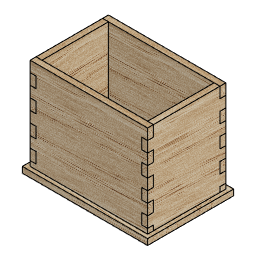
laser cut box_ (Autodesk Fusion 360 design; units mm, degrees)
Autodesk Fusion 360 part; units mm, degrees
sketch "base" plane through (0, 0, 0) normal (0, 0, 1) x (1, 0, 0) in component "base"
  line L0 (0, 0) -> (60, 0)
  line L1 (60, 0) -> (60, 40)
  line L2 (60, 40) -> (0, 40)
  line L3 (0, 40) -> (0, 0)
  line L4 (60, 20) -> (0, 20) construction
  line L5 (30, 40) -> (30, 0) construction
  line L6 (-2, 42) -> (62, 42)
  line L7 (62, 42) -> (62, -2)
  line L8 (62, -2) -> (-2, -2)
  line L9 (-2, -2) -> (-2, 42)
  line L10 (-2, 42) -> (62, -2) construction
  line L11 (62, 42) -> (-2, -2) construction
  point P0 (30, 20)
  dimension "d14" = 60
  dimension "d15" = 40
  dimension "d16" = 2
  dimension "d17" = 2
  constraint horizontal L0
  constraint vertical L1
  constraint horizontal L2
  constraint vertical L3
  constraint coincident L0.start L3.end
  constraint midpoint L1 L4.start
  constraint midpoint L3 L4.end
  constraint midpoint L2 L5.start
  constraint midpoint L0 L5.end
  constraint horizontal L6
  constraint perpendicular L6 L7
  constraint parallel L6 L8
  constraint parallel L7 L9
  constraint coincident L10 P0
  constraint coincident L11 P0
  constraint midpoint L4 P0
  measures "d14" distance of L1.end L2.end
  measures "d15" distance of L0.end L1.end
  measures "d16" distance of L2 L6
  measures "d17" distance of L1 L7
extrude "Extrude1" add sketch "base" along normal blind 3 contours L0 L1 L2 L3 | L6 L7 L8 L9 makes body 1 in component "base"
sketch "lenghttabcut" plane through (0, 0, 3) normal (0, 0, 1) x (-1, 0, 0) in component "base"
  line L0 (2, 2) -> (-62, 2)
  line L1 (-62, 2) -> (-62, -42)
  line L2 (-62, -42) -> (2, -42)
  line L3 (2, -42) -> (2, 2)
  line L4 (-5.4545, -40) -> (-10.9091, -40)
  line L5 (-10.9091, -40) -> (-10.9091, -37)
  line L6 (-10.9091, -37) -> (-5.4545, -37)
  line L7 (-5.4545, -37) -> (-5.4545, -40)
  line L8 (-60, -40) -> (0, -40)
  line L9 (0, -40) -> (0, 0)
  dimension "d20" = 5.4545
  dimension "d21" = 5.4545
  dimension "d35" = 3
  constraint horizontal L4
  constraint vertical L5
  constraint horizontal L6
  constraint vertical L7
  constraint collinear L4 L8
  measures "d20" distance of L7 L9
  measures "d21" distance of L4.start L4.end
  measures "d35" distance of L4.start L6.end
extrude "Extrude2" cut sketch "lenghttabcut" against normal blind 3 contours L4 L5 L6 L7 L8 bodies 1 in component "base"
pattern_linear "R-Pattern1" count 5 spacing 10.9091 along (1, 0, 0) of "Extrude2" in component "base"
ref_plane "WorkPlane1" through (30, 40, 1.5) normal (0, 1, 0) x (-1, 0, 0) in component "back"
sketch "back" plane through (30, 40, 1.5) normal (0, 1, 0) x (1, 0, 0) in component "back"
  line L0 (-30, 1.5) -> (30, 1.5)
  line L1 (30, 1.5) -> (30, -48.5)
  line L2 (30, -48.5) -> (-30, -48.5)
  line L3 (-30, -48.5) -> (-30, 1.5)
  point P0 (0, 1.5)
  dimension "d29" = 50
  dimension "d30" = 60
  constraint horizontal L0
  constraint vertical L1
  constraint horizontal L2
  constraint vertical L3
  constraint midpoint L0 P0
  measures "d29" distance of L0.start L2.end
  measures "d30" distance of L1.end L2.end
extrude "Extrude1'" add sketch "back" against normal blind 3 separate body makes body 2 in component "back"
sketch "heighttabcut" plane through (60, 0, 0) normal (1, 0, 0) x (0, 1, 0) in component "back"
  line L0 (40, 0) -> (40, 50)
  line L1 (40, 50) -> (37, 50)
  line L2 (37, 50) -> (37, 0)
  line L3 (37, 0) -> (40, 0)
  line L4 (37, 11.1111) -> (40, 11.1111)
  line L5 (40, 11.1111) -> (40, 5.5556)
  line L6 (40, 5.5556) -> (37, 5.5556)
  line L7 (37, 5.5556) -> (37, 11.1111)
  line L8 (42, 0) -> (-2, 0)
  dimension "d33" = 5.5556
  dimension "d34" = 5.5556
  constraint horizontal L4
  constraint vertical L5
  constraint horizontal L6
  constraint vertical L7
  constraint coincident L0 L5.end
  constraint coincident L2 L4.start
  measures "d33" distance of L6 L8
  measures "d34" distance of L4.end L5.end
combine "Combine1" operation cut target body 2 tool bodies 1 keep tools in component "back"
extrude "Extrude2'" cut sketch "heighttabcut" against normal blind 3 contours L0 L2 L4 L5 L6 L7 bodies 2 in component "back"
pattern_linear "R-Pattern1'" count 4 spacing 11.1111 along (0, 0, 1) of "Extrude2'" in component "back"
extrude "Extrude1''" add 1 faces at (28.0909, 40, 28.7778) along direction (0, 1, 0) blind 3 from surface at -40 separate body on bodies 2 makes body 3 in component "front"
combine "Combine1'" operation cut target body 1 tool bodies 3 keep tools in component "base"
sketch "widthtabcut" plane through (0, 0, 3) normal (0, 0, 1) x (-1, 0, 0) in component "base"
  line L0 (-5.4545, 0) -> (-5.4545, -3)
  line L1 (-5.4545, -3) -> (-10.9091, -3)
  line L2 (-10.9091, -3) -> (-10.9091, 0)
  line L3 (-10.9091, 0) -> (-5.4545, 0)
  line L4 (-16.3636, 0) -> (-16.3636, -3)
  line L5 (-16.3636, -3) -> (-21.8182, -3)
  line L6 (-21.8182, -3) -> (-21.8182, 0)
  line L7 (-21.8182, 0) -> (-16.3636, 0)
  line L8 (-27.2727, 0) -> (-27.2727, -3)
  line L9 (-27.2727, -3) -> (-32.7273, -3)
  line L10 (-32.7273, -3) -> (-32.7273, 0)
  line L11 (-32.7273, 0) -> (-27.2727, 0)
  line L12 (-38.1818, 0) -> (-38.1818, -3)
  line L13 (-38.1818, -3) -> (-43.6364, -3)
  line L14 (-43.6364, -3) -> (-43.6364, 0)
  line L15 (-43.6364, 0) -> (-38.1818, 0)
  line L16 (-49.0909, 0) -> (-49.0909, -3)
  line L17 (-49.0909, -3) -> (-54.5455, -3)
  line L18 (-54.5455, -3) -> (-54.5455, 0)
  line L19 (-54.5455, 0) -> (-49.0909, 0)
  line L20 (-49.0909, -37) -> (-49.0909, -40)
  line L21 (-49.0909, -40) -> (-54.5455, -40)
  line L22 (-54.5455, -40) -> (-54.5455, -37)
  line L23 (-54.5455, -37) -> (-49.0909, -37)
  line L24 (-38.1818, -37) -> (-38.1818, -40)
  line L25 (-38.1818, -40) -> (-43.6364, -40)
  line L26 (-43.6364, -40) -> (-43.6364, -37)
  line L27 (-43.6364, -37) -> (-38.1818, -37)
  line L28 (-27.2727, -37) -> (-27.2727, -40)
  line L29 (-27.2727, -40) -> (-32.7273, -40)
  line L30 (-32.7273, -40) -> (-32.7273, -37)
  line L31 (-32.7273, -37) -> (-27.2727, -37)
  line L32 (-16.3636, -37) -> (-16.3636, -40)
  line L33 (-16.3636, -40) -> (-21.8182, -40)
  line L34 (-21.8182, -40) -> (-21.8182, -37)
  line L35 (-21.8182, -37) -> (-16.3636, -37)
  line L36 (-5.4545, -37) -> (-5.4545, -40)
  line L37 (-5.4545, -40) -> (-10.9091, -40)
  line L38 (-10.9091, -40) -> (-10.9091, -37)
  line L39 (-10.9091, -37) -> (-5.4545, -37)
  line L40 (2, 2) -> (-62, 2)
  line L41 (-62, 2) -> (-62, -42)
  line L42 (-62, -42) -> (2, -42)
  line L43 (2, -42) -> (2, 2)
  line L44 (-60, -26.6667) -> (-57, -26.6667)
  line L45 (-57, -26.6667) -> (-57, -13.3333)
  line L46 (-57, -13.3333) -> (-60, -13.3333)
  line L47 (-60, -13.3333) -> (-60, -26.6667)
  line L48 (-60, -40) -> (0, -40)
  line L49 (-60, 0) -> (-60, -40)
  dimension "d45" = 3
  dimension "d46" = 13.3333
  dimension "d47" = 13.3333
  constraint horizontal L44
  constraint vertical L45
  constraint horizontal L46
  constraint vertical L47
  constraint collinear L47 L49
  measures "d45" distance of L44.start L44.end
  measures "d46" distance of L44 L48
  measures "d47" distance of L44.start L46.end
extrude "Extrude3" cut sketch "widthtabcut" against normal blind 3 contours L44 L45 L46 L47 L49 bodies 1 in component "base"
pattern_linear "R-Pattern2" count 1 spacing 0 along (0, -1, 0) of "Extrude3" in component "base"
sketch "Sketch1" plane through (60, 0, 0) normal (1, 0, 0) x (0, 1, 0) in component "right"
  line L0 (37, 44.4444) -> (40, 44.4444)
  line L1 (40, 44.4444) -> (40, 50)
  line L2 (40, 50) -> (37, 50)
  line L3 (37, 50) -> (37, 44.4444)
  line L4 (0, 0) -> (40, 0)
  line L5 (40, 0) -> (40, 50)
  line L6 (40, 50) -> (0, 50)
  line L7 (0, 50) -> (0, 0)
  constraint perpendicular L4 L5
  constraint parallel L4 L6
  constraint parallel L5 L7
  constraint horizontal L4
  constraint coincident L4.start L7.end
  constraint coincident L1.end L2.start
extrude "Extrude1'''" add sketch "Sketch1" against normal blind 3 separate body makes body 4 in component "right"
combine "Combine1''" operation cut target body 4 tool bodies 2 keep tools in component "right"
combine "Combine2" operation cut target body 4 tool bodies 3 keep tools in component "right"
combine "Combine3" operation cut target body 4 tool bodies 1 keep tools in component "right"
extrude "Extrude1''''" add 1 faces at (57, 17.7778, 12.1111) along direction (-1, 0, 0) blind 3 from surface at 54 separate body on bodies 4 makes body 5 in component "left"
combine "Combine2'" operation cut target body 2 tool bodies 5 keep tools in component "back"
combine "Combine1'''" operation cut target body 3 tool bodies 5 keep tools in component "front"
combine "Combine2''" operation cut target body 1 tool bodies 5 keep tools in component "base"
component "base" placed x (1, 0, 0) y (0, 1, 0) z (0, 0, 1) at (0, 0, 0)
component "back" placed x (1, 0, 0) y (0, 1, 0) z (0, 0, 1) at (0, 0, 0)
component "front" placed x (1, 0, 0) y (0, 1, 0) z (0, 0, 1) at (0, 0, 0)
component "right" placed x (1, 0, 0) y (0, 1, 0) z (0, 0, 1) at (0, 0, 0)
component "left" placed x (1, 0, 0) y (0, 1, 0) z (0, 0, 1) at (0, 0, 0)
equation "length = 60 mm" comment "exterior"
equation "width = 40 mm" comment "exterior"
equation "height = 50 mm" comment "exterior"
equation "thick = 3 mm" comment "material thickness"
equation "Ltab = 5" comment "No. tab"
equation "Wtab = 1" comment "No. tab"
equation "Htab = 4" comment "No. tab"
equation "WtabWidth = width / ( ( Wtab * 2 ) + 1 )" comment "tab size"
equation "LtabWidth = length / ( ( Ltab * 2 ) + 1 )" comment "tab size"
equation "HtabWidth = height / ( ( Htab * 2 ) + 1 )" comment "tab size"
equation "baseoffset = 2 mm" comment "Base outline"
equation "d14 = length"
equation "d15 = width"
equation "d16 = baseoffset"
equation "d17 = baseoffset"
equation "d18 = thick"
equation "d20 = LtabWidth"
equation "d21 = LtabWidth"
equation "d22 = -thick"
equation "d24 = Ltab"
equation "d26 = length - LtabWidth * 3"
equation "d28 = -baseoffset"
equation "d29 = height"
equation "d30 = length"
equation "d31 = -thick"
equation "d33 = HtabWidth"
equation "d34 = HtabWidth"
equation "d35 = thick"
equation "d36 = -thick"
equation "d38 = Htab"
equation "d40 = height - HtabWidth * 3"
equation "d42 = -baseoffset"
equation "d43 = thick"
equation "d45 = thick"
equation "d46 = WtabWidth"
equation "d47 = WtabWidth"
equation "d48 = -thick"
equation "d50 = Wtab"
equation "d52 = width - WtabWidth * 3"
equation "d54 = -thick"
equation "d56 = -baseoffset - thick"
equation "d57 = thick"
